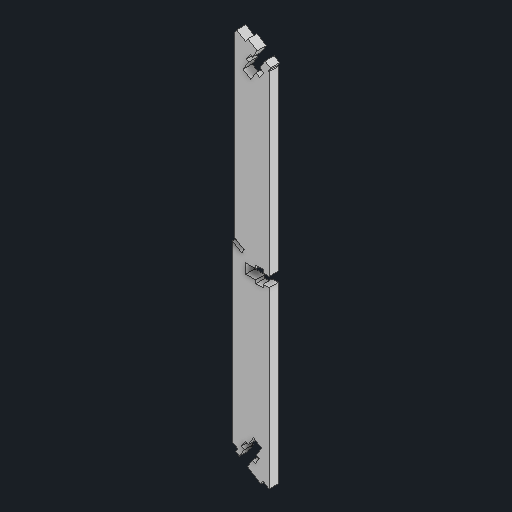
# Autodesk Inventor part: Inner Bracket
Saved by Autodesk Inventor 2023 (Build 270158000, 158)
## iProperties
Created: 2022-06-20
Part Number: Inner Bracket
Material: Generic
Document SubType Name: Modeling
Designer: FizzyApple12
Density: 1 g/cm^3
Appearance: Default
Author: FizzyApple12
Autodesk Inventor part; units mm, degrees
ref_plane "YZ Plane" through (0, 0, 0) normal (1, 0, 0) x (0, 1, 0)
ref_plane "XZ Plane" through (0, 0, 0) normal (0, 1, 0) x (-1, 0, 0)
ref_plane "XY Plane" through (0, 0, 0) normal (0, 0, 1) x (1, 0, 0)
ref_plane "Work Plane1" through (0, 0, 0) normal (0, 0, 1) x (1, 0, 0)
sketch "Sketch1" plane through (0, 0, 0) normal (0, 0, 1) x (1, 0, 0)
  line L0 (-13.9399, 12.3161) -> (-5.7696, 7.2832) projected
  line L1 (-15.6051, 9.6128) -> (-13.9399, 12.3161) projected
  line L2 (-7.4348, 4.5799) -> (-15.6051, 9.6128) projected
  line L3 (-5.7696, 7.2832) -> (-7.4348, 4.5799) construction
  line L4 (-5.4698, 3.3694) -> (-7.4348, 4.5799) construction
  line L5 (-3.8046, 6.0727) -> (1.6652, 2.7033) projected
  line L6 (-5.4698, 3.3694) -> (-3.8046, 6.0727) construction
  line L7 (0, 0) -> (-5.4698, 3.3694) projected
  line L8 (0, 0) -> (1.6652, 2.7033) projected
  line L9 (-5.3472, -249.9446) -> (-16.3579, -243.162) projected
  line L10 (-14.6927, -240.4587) -> (-3.682, -247.2413) projected
  line L11 (-16.3579, -243.162) -> (-14.6927, -240.4587) construction
  line L12 (-9.0019, -247.6933) -> (-20.2167, -240.7849) construction
  line L13 (-6.6483, -245.4141) -> (-18.5515, -238.0817) construction
  line L14 (0.5444, -249.8448) -> (0.5444, -249.8448) projected
  line L15 (0.5444, -2.2912) -> (0.5444, 0.8838) construction
  line L16 (0.5444, 0.8838) -> (0.5444, 0.8838) construction
  line L17 (0.5444, 0.8838) -> (0.5444, -253.0198) construction
  line L18 (0.5444, -253.0198) -> (0.5444, -253.0198) construction
  line L19 (0.5444, -253.0198) -> (0.5444, 0.8838) construction
  line L20 (0.5444, 0.8838) -> (0.5444, 0.8838) construction
  line L21 (0.5444, 0.8838) -> (0.5444, -2.2912) construction
  line L22 (0.5444, -2.2912) -> (0.5444, -2.2912) construction
  line L23 (-7.4904, 8.3432) -> (-9.1556, 5.6399)
  line L24 (-3.7491, 2.3094) -> (-2.0838, 5.0127)
  line L25 (0, 0) -> (0.5444, -0.3354)
  line L26 (0.5444, -0.3354) -> (0.5444, -253.0198)
  line L27 (-12.9719, -241.5187) -> (-14.6371, -244.222)
  line L28 (-15.6051, 9.6128) -> (-23.1742, 14.2754)
  line L29 (-23.1742, 14.2754) -> (-23.1742, -111.4572)
  line L30 (-25.9909, -237.228) -> (-24.3256, -234.5248) construction
  line L31 (-21.0892, -112.7416) -> (-23.1742, -111.4572) construction
  line L32 (-23.1742, -111.4572) -> (0.5444, -126.068) construction
  line L33 (-23.1742, -111.4572) -> (-24.8395, -114.1605) construction
  line L34 (-22.7544, -115.4449) -> (-24.8395, -114.1605) construction
  line L35 (-24.8395, -114.1605) -> (0.5444, -129.797) construction
  line L36 (-24.8395, -114.1605) -> (-24.8395, -234.2082)
  line L37 (-24.3256, -234.5248) -> (-24.8395, -234.2082) construction
  line L38 (-24.8395, -234.2082) -> (-18.5515, -238.0817)
  line L39 (-12.9719, -241.5187) -> (-4.6458, -228.0024)
  line L40 (-18.5515, -238.0817) -> (-10.2253, -224.5653)
  line L41 (-10.2253, -224.5653) -> (-4.6458, -228.0024)
  line L42 (-14.4373, -243.8976) -> (-5.1474, -249.6202)
  line L43 (1.4654, 2.3789) -> (-2.2837, 4.6883)
  line L44 (-7.6902, 8.0188) -> (-14.1397, 11.9917)
  line L45 (0.5444, -122.6898) -> (3.3735, -122.6898) construction
  line L46 (0.5444, -129.4462) -> (3.3735, -129.4462) construction
  line L47 (-3.7491, 2.3094) -> (-12.0752, -11.2069)
  line L48 (-12.0752, -11.2069) -> (-17.4817, -7.8765)
  line L49 (-17.4817, -7.8765) -> (-9.1556, 5.6399)
  line L50 (-14.7785, -9.5417) -> (-3.6876, 6.0006) construction
  line L51 (-15.2312, -0.6107) -> (-6.1856, -7.0655)
  line L52 (-6.1856, -7.0655) -> (-3.2348, -2.9304)
  line L53 (-3.2348, -2.9304) -> (-12.2804, 3.5245)
  line L54 (-12.2804, 3.5245) -> (-15.2312, -0.6107)
  line L55 (-15.2312, -0.6107) -> (-3.2348, -2.9304) construction
  line L56 (-6.1856, -7.0655) -> (-12.2804, 3.5245) construction
  line L57 (-7.4356, -226.2838) -> (-17.4269, -242.5035) construction
  line L58 (-18.4941, -233.6421) -> (-9.0327, -239.4704)
  line L59 (-9.0327, -239.4704) -> (-6.3683, -235.1452)
  line L60 (-6.3683, -235.1452) -> (-15.8298, -229.3169)
  line L61 (-15.8298, -229.3169) -> (-18.4941, -233.6421)
  line L62 (-18.4941, -233.6421) -> (-6.3683, -235.1452) construction
  line L63 (-9.0327, -239.4704) -> (-15.8298, -229.3169) construction
  line L64 (0.5444, -122.6898) -> (-15.6765, -122.6898)
  line L65 (-15.6765, -122.6898) -> (-15.6765, -129.4462)
  line L66 (-15.6765, -129.4462) -> (0.5444, -129.4462)
  line L67 (3.3735, -126.068) -> (-15.6765, -126.068) construction
  line L68 (-8.6915, -131.6242) -> (-8.6915, -120.5117)
  line L69 (-8.6915, -120.5117) -> (-3.6115, -120.5117)
  line L70 (-3.6115, -120.5117) -> (-3.6115, -131.6242)
  line L71 (-3.6115, -131.6242) -> (-8.6915, -131.6242)
  line L72 (-8.6915, -131.6242) -> (-3.6115, -120.5117) construction
  line L73 (-8.6915, -120.5117) -> (-3.6115, -131.6242) construction
  line L74 (-24.8395, -114.1605) -> (-10.9932, -122.6898)
  line L75 (-23.1742, -111.4572) -> (-8.4754, -120.5117)
  line L76 (-16.6864, -115.4537) -> (-18.3516, -118.157)
  line L77 (-20.1943, 16.1688) -> (-21.8595, 13.4656) construction
  line L78 (-21.8595, 13.4656) -> (-23.1742, 11.3313)
  line L79 (-23.2443, -111.414) -> (-24.9095, -114.1173) projected
  line L80 (-3.6115, -131.6242) -> (0.5444, -131.6242)
  line L81 (-3.6115, -120.5117) -> (0.5444, -120.5117)
  line L82 (-3.682, -247.2413) -> (0.5444, -249.8448)
  line L83 (-5.3472, -249.9446) -> (-3.682, -247.2413) projected
  line L84 (-22.6481, -239.2872) -> (-20.9829, -236.5839) projected
  line L85 (-18.3229, -241.9515) -> (-22.6481, -239.2872) projected
  line L86 (-18.5515, -238.0817) -> (-20.2167, -240.7849)
  line L87 (-20.0168, -240.4606) -> (-22.4483, -238.9628)
  line L88 (0.5444, -122.6898) -> (0.5444, -129.4462) projected
  line L89 (0.5444, -122.6898) -> (0.5444, -129.4462) projected
  line L90 (3.3735, -122.6898) -> (3.3735, -129.4462) projected
  line L91 (-2.79, 5.4477) -> (-4.5852, 6.5535) projected
  point P0 (-6.4523, 3.9747)
  point P1 (-9.233, -1.7705)
  point P2 (-12.4312, -234.3936)
  point P3 (-6.1515, -126.068)
  point P4 (-16.5532, -234.8378)
  point P5 (-13.8888, -230.5125)
  point P6 (-8.3093, -233.9495)
  point P7 (-10.9736, -238.2748)
  point P8 (0.5444, -129.4462)
  point P9 (-3.6115, -129.4462)
  point P10 (-8.6915, -129.4462)
  point P11 (-8.6915, -122.6898)
  point P12 (-3.6115, -122.6898)
  point P13 (0.5444, -122.6898)
  point P14 (-5.8342, -1.0755)
  point P15 (-8.5047, -5.4107)
  point P16 (-13.6854, -1.7137)
  point P17 (-11.015, 2.6214)
  dimension "d0" = 3.175
  dimension "d1" = 3.175
  dimension "d2" = 2.021
  dimension "d3" = 2.021
  dimension "d5" = 19.05
  dimension "d7" = 0.381
  dimension "d8" = 0.381
  dimension "d10" = 8.89
  dimension "d11" = 11.1125
  dimension "d12" = 5.08
  dimension "d13" = 11.1125
  dimension "d14" = 5.08
  dimension "d15" = 19.05
  dimension "d16" = 11.1125
  dimension "d17" = 5.08
  dimension "d18" = 7.62
  dimension "d21" = 0.381
  dimension "d22" = 19.05
  constraints: 122 end point, 29 point on line, 19 perpendicular, 15 parallel, 14 midpoint, 12 collinear, 2 horizontal, 4 other
  measures "d0" distance from line of point (-6.452, 3.975) L24
  measures "d1" distance from line of L23 point (-6.452, 3.975)
  measures "d2" distance between parallel lines of L6 L24
  measures "d3" distance between parallel lines of L11 L27
  measures "d5" distance between parallel lines of L12 L41
  measures "d7" distance between parallel lines of L9 L42
  measures "d8" distance between parallel lines of L0 L44
  measures "d10" distance from line of L28.end L1
  measures "d11" distance of L51.start L51.end
  measures "d12" distance of L52.end L51.end
  measures "d13" distance of L58.start L58.end
  measures "d14" distance of L59.end L58.end
  measures "d15" distance from line of L67.start L65
  measures "d16" distance of L68.start L68.end
  measures "d17" distance of L68.end L69.end
  measures "d18" distance between parallel lines of L33 L76
  measures "d21" distance between parallel lines of L85 L87
  measures "d22" distance between parallel lines of L48 L0
extrude "Extrusion1" add sketch "Sketch1" along normal blind 6.35 contours L44 L23 L2 L1 | L2 L49 L53 L54 L51 L48 L47 L52 L7 L25 L26 L81 L69 L75 L29 L78 L28 | L24 L43 L8 L7 | L75 L69 L68 L64 L74 L76 | L74 L64 L65 L66 L68 L71 L80 L26 L82 L10 L39 L58 L59 L60 L41 L40 L61 L38 L36 | L81 L26 L64 L70 | L66 L26 L80 L70 | L38 L86 L87 L84 | L83 L42 L27 L10
equation "\"d1\" = d0"
equation "\"d3\" = d2"
body "Solid1"
